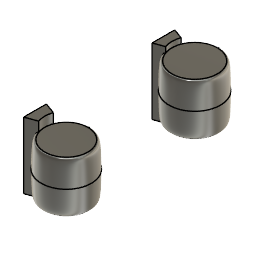
fork-upper-crown30-type-af7mm-fox38-miran (Autodesk Fusion 360 archive; units mm, degrees)
design "Untitled"
part number: 2026-04-06-17-23-14-010
part number: 2026-04-07-10-34-04-831
Autodesk Fusion 360 part; units mm, degrees
sketch "Fox 36" plane through (0, 0, 0) normal (1, 0, 0) x (0, 1, 0)
  line L0 (0, 0) -> (0, 45.8)
  line L1 (0, 45.8) -> (19.45, 45.8)
  line L2 (0, 43.65) -> (21.6, 43.65) construction
  line L3 (0, 2.15) -> (21.6, 2.15) construction
  line L4 (0, 0) -> (19.45, 0)
  line L5 (0, 22.9) -> (22.6, 22.9) construction
  spline S0 degree 5 poles (19.45, 0) (19.6516, 0) (20.0375, 0.0457) (20.5637, 0.25) (21.1485, 0.7925) (21.6357, 1.9079) (21.9282, 3.7985) (22.1323, 6.7357) (22.286, 10.4562) (22.414, 14.5267) (22.517, 18.3729) (22.5731, 20.8212) (22.5951, 22.1006) (22.6, 22.6793) (22.6, 22.9) knots 0 0 0 0 0 0 0.1 0.2 0.3 0.4 0.5 0.6 0.7 0.8 0.9 1 1 1 1 1 1
  line L6 (17.2748, 0) -> (21.6252, 0)
  line L7 (22.6, 21.9821) -> (22.6, 23.8179)
  line L8 (21.2003, 0.5604) -> (21.9997, 3.7396)
  spline S1 degree 5 poles (19.45, 45.8) (19.6516, 45.8) (20.0375, 45.7543) (20.5637, 45.55) (21.1485, 45.0075) (21.6357, 43.8921) (21.9282, 42.0015) (22.1323, 39.0643) (22.286, 35.3438) (22.414, 31.2733) (22.517, 27.4271) (22.5731, 24.9788) (22.5951, 23.6994) (22.6, 23.1207) (22.6, 22.9) knots 0 0 0 0 0 0 0.1 0.2 0.3 0.4 0.5 0.6 0.7 0.8 0.9 1 1 1 1 1 1
  line L9 (17.2748, 45.8) -> (21.6252, 45.8)
  line L10 (21.2003, 45.2396) -> (21.9997, 42.0604)
  line L11 (22.6, 23.8179) -> (22.6, 21.9821)
  point P0 (0, 2.15)
  point P1 (0, 43.65)
  point P2 (21.6, 43.65)
  dimension "d1" = 45.8
  dimension "d2" = 41.5
  dimension "d3" = 2.15
  dimension "d4" = 22.6
  dimension "d5" = 21.6
  dimension "d6" = 21.6
  dimension "d7" = 19.45
  dimension "d8" = 19.45
  constraint coincident L0.start L4.start
  constraint vertical L0
  constraint coincident L0 P0
  constraint coincident L0 P1
  constraint perpendicular L0 L1
  constraint coincident P1 L2.start
  constraint perpendicular L0 L2
  constraint coincident P0 L3.start
  constraint perpendicular L0 L3
  constraint perpendicular L0 L4
  constraint midpoint L0 L5.start
  constraint perpendicular L0 L5
  constraint midpoint L4.end L6
  constraint horizontal L6
  constraint midpoint L5.end L7
  constraint vertical L7
  constraint midpoint L3.end L8
  constraint symmetric L3.end L5 P2
  constraint symmetric L4.end L5 L1.end
  constraint symmetric S0.end L5 S1.end
  constraint symmetric L5 L6.start L9.start
  constraint symmetric L5 L6.end L9.end
  constraint symmetric L5 L7.start L7.end
  constraint symmetric L5 L7.end L7.start
  constraint symmetric L5 L8.start L10.start
  constraint symmetric L5 L8.end L10.end
  measures "d1" distance of L0.start L0.end
  measures "d2" distance of P0 P1
  measures "d3" distance of L0.end P1
  measures "d4" distance of L5.start L5.end
  measures "d5" distance of P1 P2
  measures "d6" distance of P0 L3.end
  measures "d7" distance of L0.end L1.end
  measures "d8" distance of L0.start L4.end
sketch "Fox 38" plane through (0, 0, 0) normal (1, 0, 0) x (0, 1, 0)
  line L0 (116.1014, 49.5016) -> (136.6014, 49.5016)
  line L1 (116.1014, 3.2016) -> (136.6014, 3.2016)
  spline S0 degree 5 poles (136.6014, 3.2016) (136.7867, 3.2016) (137.1382, 3.2369) (137.6079, 3.3945) (138.1194, 3.8534) (138.5722, 5.0072) (138.8725, 7.0893) (139.065, 10.1804) (139.1811, 13.9894) (139.2474, 18.0687) (139.2825, 21.8765) (139.2958, 24.2872) (139.3004, 25.5521) (139.3014, 26.1294) (139.3014, 26.3516) knots 0 0 0 0 0 0 0.1 0.2 0.3 0.4 0.5 0.6 0.7 0.8 0.9 1 1 1 1 1 1
  line L2 (134.4263, 3.2016) -> (138.7766, 3.2016)
  line L3 (138.1017, 3.5121) -> (138.9012, 6.6912)
  line L4 (139.3014, 25.4337) -> (139.3014, 27.2695)
  line L5 (116.1014, 3.2016) -> (116.1014, 49.5016)
  line L6 (116.1014, 26.3516) -> (139.3014, 26.3516) construction
  line L7 (116.1014, 5.1016) -> (138.5014, 5.1016) construction
  spline S1 degree 5 poles (136.6014, 49.5016) (136.7867, 49.5016) (137.1382, 49.4664) (137.6079, 49.3088) (138.1194, 48.8498) (138.5722, 47.6961) (138.8725, 45.6139) (139.065, 42.5229) (139.1811, 38.7139) (139.2474, 34.6346) (139.2825, 30.8267) (139.2958, 28.416) (139.3004, 27.1512) (139.3014, 26.5738) (139.3014, 26.3516) knots 0 0 0 0 0 0 0.1 0.2 0.3 0.4 0.5 0.6 0.7 0.8 0.9 1 1 1 1 1 1
  line L8 (134.4263, 49.5016) -> (138.7766, 49.5016)
  line L9 (138.1017, 49.1912) -> (138.9012, 46.0121)
  line L10 (139.3014, 27.2695) -> (139.3014, 25.4337)
  line L11 (116.1014, 47.6016) -> (138.5014, 47.6016) construction
  point P0 (116.1014, 3.2016)
  point P1 (138.5014, 47.6016)
  point P2 (116.1014, 5.1016)
  point P3 (116.1014, 47.6016)
  dimension "d10" = 46.3
  dimension "d11" = 42.5
  dimension "d12" = 1.9
  dimension "d13" = 23.2
  dimension "d14" = 22.4
  dimension "d15" = 22.4
  dimension "d16" = 20.5
  dimension "d17" = 20.5
  constraint coincident P0 L1.start
  constraint vertical L5
  constraint coincident P2 L5
  constraint coincident P3 L5
  constraint perpendicular L0 L5
  constraint coincident P3 L11.start
  constraint perpendicular L5 L11
  constraint coincident L7.start P2
  constraint perpendicular L5 L7
  constraint perpendicular L1 L5
  constraint midpoint L6.start L5
  constraint perpendicular L5 L6
  constraint midpoint L1.end L2
  constraint horizontal L2
  constraint midpoint S0.end L4
  constraint vertical L4
  constraint midpoint L7.end L3
  constraint symmetric L7.end L11.end L6
  constraint symmetric L1.end L0.end L6
  constraint symmetric S0.end S1.end L6
  constraint symmetric L8.start L2.start L6
  constraint symmetric L8.end L2.end L6
  constraint symmetric L4.end L4.start L6
  constraint symmetric L4.start L4.end L6
  constraint symmetric L3.start L9.start L6
  constraint symmetric L3.end L9.end L6
  measures "d10" distance of P0 L0.start
  measures "d11" distance of P2 P3
  measures "d12" distance of L0.start P3
  measures "d13" distance of L6.start S0.end
  measures "d14" distance of P1 P3
  measures "d15" distance of L7.end L7.start
  measures "d16" distance of L0.start L0.end
  measures "d17" distance of L1.end P0
revolve "Revolve1" add sketch "Fox 36" angle 360 about axis through (0, 0, 0) along (0, 0, 1) makes body 1
revolve "Revolve2" add sketch "Fox 38" angle 360 about axis through (0, 116.1014, 3.2016) along (0, 0, 1) separate body makes body 2
ref_plane "WorkPlane1" through (0, 116.1014, 54.5016) normal (0, 0, 1) x (1, 0, 0)
sketch "Sketch3" plane through (0, 0, 54.5016) normal (0, 0, 1) x (1, 0, 0)
  circle A0 centre (0, 116.1014) radius 20.5
  circle A1 centre (0, 0) radius 19.45
  line L0 (0, 0) -> (-57.1658, -20.8066)
  line L1 (0, 0) -> (61.3002, 0) construction
  line L2 (0, 0) -> (-55.3132, 20.1324)
  line L3 (0, 0) -> (59.3136, 0) construction
  line L4 (0, 116.1014) -> (-56.3255, 95.6006)
  line L5 (0, 116.1014) -> (60.3991, 116.1014) construction
  line L6 (0, 116.1014) -> (-42.256, 131.4814)
  line L7 (0, 116.1014) -> (45.3121, 116.1014) construction
  circle A2 centre (0, 116.1014) radius 23.2
  circle A3 centre (0, 0) radius 22.6
  line L8 (-28.3166, 136.3446) -> (-28.3166, -27.6887)
  dimension "d21" = 160
  dimension "d22" = 160
  dimension "d23" = 160
  dimension "d24" = 160
  constraint horizontal L1
  constraint coincident A1.centre L0.start
  constraint horizontal L3
  constraint horizontal L5
  constraint coincident A0.centre L4.start
  constraint horizontal L7
  constraint vertical L8
  measures "d21" angle of L0 L1
  measures "d22" angle of L2 L3
  measures "d23" angle of L4 L5
  measures "d24" angle of L6 L7
extrude "Extrude1" add sketch "Sketch3" against normal blind 60 separate body contours A0 L4 L6 A2 | L4 L6 A2 L8 | A1 L0 L2 A3 | L0 L2 A3 L8 picked at (-21.5153, 110.4279) picked at (-20.5401, 6.3603) makes body 3 at (-28.3166, 3.4355, 34.5016) makes body 4 at (-28.3166, 119.5369, 14.5016)
combine "Combine1" operation cut target body 3 tool bodies 1 keep tools
combine "Combine2" operation cut target body 4 tool bodies 2 keep tools
sketch "Sketch4" plane through (-28.3166, 0, 0) normal (-1, 0, 0) x (0, -1, 0)
  line L0 (10.3064, 54.5016) -> (-10.3064, 54.5016)
  line L1 (-10.3064, 54.5016) -> (-10.3064, -5.4984)
  line L2 (-10.3064, -5.4984) -> (10.3064, -5.4984)
  line L3 (10.3064, -5.4984) -> (10.3064, 54.5016)
  line L4 (6.486, 53.8022) -> (-10.3064, 54.5016) construction
  line L5 (-10.3064, 54.5016) -> (-12.2934, 6.7948) construction
  line L6 (-12.2934, 6.7948) -> (4.499, 6.0954) construction
  line L7 (4.499, 6.0954) -> (6.486, 53.8022) construction
  line L8 (-7.7297, 22.9) -> (7.7297, 22.9)
  line L9 (-111.3811, 54.5856) -> (-131.3486, 54.5016) construction
  line L10 (-131.3486, 54.5016) -> (-131.1416, 5.259) construction
  line L11 (-131.1416, 5.259) -> (-111.1741, 5.3429) construction
  line L12 (-111.1741, 5.3429) -> (-111.3811, 54.5856) construction
  dimension "d27" = 10
  dimension "d28" = 0
  dimension "d29" = 10
  text T0 "36" font "Arial" height 10 bold align left top in box 16.807 x 47.7482 at (6.486, 53.8022) x (-0.999134, 0.041614) y (-0.041614, -0.999134) spacing 1 kerned
  text T1 "38\n" font "Arial" height 10 bold align left top in box 19.9677 x 49.2431 at (-111.3811, 54.5856) x (-0.999991, -0.004203) y (0.004203, -0.999991) spacing 1 kerned
  constraint coincident L0.end
extrude "Extrude2" cut sketch "Sketch4" against normal blind 1 text T1 T0 bodies 3 4
copy_body "Body->Comp1" bodies 1 removing the originals makes body 5 in component "36 POS"
component "36 POS" placed x (1, 0, 0) y (0, 1, 0) z (0, 0, 1) at (0, 0, 0)
equation "d3 = ( d1 - d2 ) / 2"
equation "d6 = d5"
equation "d7 = d5 - d3"
equation "d8 = d6 - d3"
equation "d12 = ( d10 - d11 ) / 2"
equation "d15 = d14"
equation "d16 = d14 - d12"
equation "d17 = d16"
equation "d21 = d24"
equation "d22 = d24"
equation "d23 = d24"
equation "d28 = '36'"
equation "d30 = '38 '"
named bodies: "36 POS", "38 POS", "36 NEG", "38 NEG"
